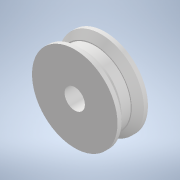
# Autodesk Inventor part: koło_pasowe_duze
Saved by Autodesk Inventor 2022.3 (Build 263350000, 350)
## iProperties
Created: 2022-12-14
Part Number: koło_pasowe_duze
Material: Generic
Document SubType Name: Modeling
Designer: komputer
Density: 1 g/cm^3
Appearance: Default
Author: komputer
Autodesk Inventor part; units mm, degrees
ref_plane "YZ Plane" through (0, 0, 0) normal (1, 0, 0) x (0, 1, 0)
ref_plane "XZ Plane" through (0, 0, 0) normal (0, 1, 0) x (-1, 0, 0)
sketch "Sketch1" plane through (0, 0, 0) normal (0, 0, 1) x (1, 0, 0)
  line L0 (7.011, 4.2884) -> (7.2242, 4.5036)
  line L1 (9.7459, 1.5804) -> (9.5018, 1.4012)
  line L2 (10.4101, 2.9001) -> (10.3642, 2.6007)
  line L3 (6.7053, 2.2945) -> (6.6103, 2.5821)
  line L4 (9.2149, 4.8291) -> (9.4855, 4.6929)
  circle A0 centre (8.485, 3.042) radius 1
  circle A1 centre (8.485, 3.042) radius 1.9244
  circle A2 centre (0, 0) radius 4.2028
  circle A3 centre (0, 0) radius 1
extrude "Extrusion1" add sketch "Sketch1" against normal blind 1 contours A2
sketch "Sketch2" plane through (0, 0, -1) normal (0, 0, -1) x (-1, 0, 0)
  circle A0 centre (0, 0) radius 4.2028 projected
  circle A1 centre (0, 0) radius 1 projected
  line L0 (-6.5615, 2.8811) -> (-6.56, 3.184) projected
  line L1 (-9.4855, 4.6929) -> (-9.7314, 4.516) projected
  line L2 (-8.945, 1.1673) -> (-8.646, 1.1184) projected
  circle A2 centre (-8.485, 3.042) radius 1 projected
  circle A3 centre (-8.485, 3.042) radius 1.9485
  circle A4 centre (0, 0) radius 3.5115
  constraints: 2 centre point, 2 coincident
extrude "Extrusion2" add sketch "Sketch2" along normal blind 1 contours A4
sketch "Sketch3" plane through (0, 0, -2) normal (0, 0, -1) x (-1, 0, 0)
  circle A0 centre (0, 0) radius 4.2028 projected
  circle A1 centre (0, 0) radius 1 projected
  circle A2 centre (0, 0) radius 1 projected
ref_plane "Work Plane1" through (5.485, 0.042, -3) normal (0, 0, -1) x (0, 1, 0)
extrude "Extrusion3" add sketch "Sketch3" along normal up to surface (1 mm away)
chamfer "Chamfer1" distance 0.6 angle 45 2 edges at (4.2028, 0, -2) (-4.2028, 0, -1)
body "Solid1"
